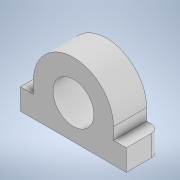
# Autodesk Inventor part: Recoil Spring Mount v1.0
Saved by Autodesk Inventor 2020 (Build 240168000, 168)
## iProperties
Created: 2021-10-29
Part Number: Recoil Spring Mount v1.0
Material: Generic
Document SubType Name: Modeling
Designer: kyle
Density: 1 g/cm^3
Appearance: Default
Author: kyle
Autodesk Inventor part; units mm, degrees
ref_plane "YZ Plane" through (0, 0, 0) normal (1, 0, 0) x (0, 1, 0)
ref_plane "XZ Plane" through (0, 0, 0) normal (0, 1, 0) x (-1, 0, 0)
ref_plane "XY Plane" through (0, 0, 0) normal (0, 0, 1) x (1, 0, 0)
sketch "Sketch1" plane through (0, 0, 0) normal (0, 0, 1) x (1, 0, 0)
  line L0 (0, 0) -> (0, 3.85)
  line L1 (0, 0) -> (19.15, 0)
  line L2 (19.15, 0) -> (19.15, 3.85)
  line L3 (0, 3.85) -> (2.325, 3.85)
  line L4 (2.325, 3.85) -> (2.325, 6)
  line L5 (19.15, 3.85) -> (16.825, 3.85)
  line L6 (16.825, 3.85) -> (16.825, 6)
  arc A0 (16.825, 6) -> (2.325, 6) centre (9.575, 6) ccw
  circle A1 centre (9.575, 6.12) radius 3.7
  point P0 (9.575, 13.25)
  dimension "d0" = 19.15
  dimension "d1" = 3.85
  dimension "d2" = 3.85
  dimension "d3" = 9.575
  dimension "d4" = 13.25
  dimension "d5" = 7.25
  dimension "d6" = 7.25
  dimension "d7" = 7.25
  dimension "d8" = 7.25
  dimension "d9" = 9.575
  dimension "d10" = 7.4
  dimension "d11" = 7.13
  constraints: 14 end point, 3 horizontal, 3 perpendicular, 3 point on circle, 2 centre point, 1 vertical
  measures "d0" distance of L0.start L1.end
  measures "d1" distance of L0.start L0.end
  measures "d2" distance of L1.end L2.end
  measures "d3" distance from line of point (9.575, 13.25) L0
  measures "d4" distance from line of L1 point (9.575, 13.25)
  measures "d5" horizontal distance of L4.end point (9.575, 13.25)
  measures "d6" horizontal distance of L6.end point (9.575, 13.25)
  measures "d7" horizontal distance of L4.end point (9.575, 13.25)
  measures "d8" horizontal distance of L6.end point (9.575, 13.25)
  measures "d9" distance from line of L0 A1.centre
  measures "d10" diameter of A1
  measures "d11" distance of A1.centre point (9.575, 13.25)
extrude "Extrusion1" add sketch "Sketch1" along normal blind 6
fillet "Fillet1" radius 1.5 2 edges at (19.15, 1.925, 0) (0, 1.925, 0)
equation "\"d2\" = d1"
equation "\"d3\" = 0.5 * d0"
equation "\"d6\" = d5"
equation "\"d7\" = d5"
equation "\"d8\" = d5"
equation "\"d9\" = d3"
body "Solid1"
